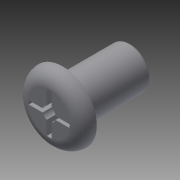
# Autodesk Inventor part: screw
Saved by Autodesk Inventor 2015 SP2 (Build 190223200, 223)
## iProperties
Created: 2016-09-05
Part Number: screw
Material: Generic
Document SubType Name: Modeling
Designer: jm799
Density: 1 g/cm^3
Appearance: Default
Author: jm799
Autodesk Inventor part; units mm, degrees
ref_plane "YZ Plane" through (0, 0, 0) normal (1, 0, 0) x (0, 1, 0)
ref_plane "XZ Plane" through (0, 0, 0) normal (0, 1, 0) x (-1, 0, 0)
ref_plane "XY Plane" through (0, 0, 0) normal (0, 0, 1) x (1, 0, 0)
sketch "Sketch1" plane through (0, 0, 0) normal (0, 1, 0) x (-1, 0, 0)
  circle A0 centre (0, 0) radius 2.5
  circle A1 centre (0, 0) radius 1.5
  dimension "d0" = 5
  dimension "d1" = 3
  constraints: 2 centre point, 2 coincident
  measures "d0" diameter of A0
  measures "d1" diameter of A1
extrude "Extrusion1" add sketch "Sketch1" along normal blind 1
sketch "Sketch2" plane through (0, 1, 0) normal (0, 1, 0) x (1, 0, 0)
  circle A0 centre (0, 0) radius 1.5
  dimension "d4" = 3
  constraints: 1 centre point, 1 coincident
  measures "d4" diameter of A0
extrude "Extrusion2" add sketch "Sketch2" along normal blind 5 and the other way blind 1
sketch "Sketch4" plane through (0, 0, 0) normal (0, -1, 0) x (1, 0, 0)
  circle A0 centre (0, 0) radius 1.5 projected
  line L0 (-0.1651, 0.1041) -> (-0.1651, 1.4909)
  line L1 (0.1791, 0.0776) -> (0.1791, 1.4893)
  line L2 (-0.1651, -0.1651) -> (-0.1651, -1.4909)
  line L3 (0.1791, -0.0776) -> (0.1791, -1.4893)
  line L4 (-0.1651, -0.1651) -> (-1.4909, -0.1651)
  line L5 (0.1791, -0.1651) -> (1.4909, -0.1651)
  line L6 (-0.1651, 0.1041) -> (-1.4964, 0.1041)
  line L7 (0.1791, 0.0776) -> (1.498, 0.0776)
  circle A1 centre (0, 0) radius 0.4994
  constraints: 16 end point, 7 point on line, 2 perpendicular, 1 centre point, 1 coincident, 1 horizontal, 1 parallel, 9 other
extrude "Extrusion4" cut sketch "Sketch4" against normal blind 1 contours A0 L5 A1 L7 | L1 A1 L0 A0 | A1 L5 L3 L2 L4 L6 L0 L1 L7 | L7 L1 A1 | A0 L2 A1 L3 | A1 L3 L5 | L6 A1 L4 A0 | L0 L6 A1 | A1 L4 L2
fillet "Fillet1" radius 1 1 edges at (2.5, 0, 0)
fillet "Fillet2" radius 0.2 1 edges at (-1.5, 6, 0)
sketch "Sketch5" plane through (0, 1, 0) normal (0, 1, 0) x (1, 0, 0)
  circle A0 centre (0, 0) radius 1.9093
  constraints: 1 centre point, 1 coincident
extrude "Extrusion5" add sketch "Sketch5" along normal blind 0.1
body "Solid1"
